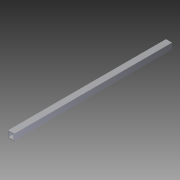
# Autodesk Inventor part: AB1-16-26-001
Saved by Autodesk Inventor 2011 SP1 (Build 150282100, 282)
## iProperties
Created: 2011-01-11
Part Number: AB1-16-26-001
Document SubType Name: Modeling
Designer: 12416547
Density: 1 g/cm^3
Author: 12416547
Autodesk Inventor part; units mm, degrees
ref_plane "YZ Plane" through (0, 0, 0) normal (1, 0, 0) x (0, 1, 0)
ref_plane "XZ Plane" through (0, 0, 0) normal (0, 1, 0) x (-1, 0, 0)
ref_plane "XY Plane" through (0, 0, 0) normal (0, 0, 1) x (1, 0, 0)
sketch "Sketch1" plane through (0, 0, 0) normal (0, 0, 1) x (1, 0, 0)
  line L0 (-24.2455, 20.5231) -> (1.1545, 20.5231)
  line L1 (1.1545, 20.5231) -> (1.1545, -4.8769)
  line L2 (1.1545, -4.8769) -> (-24.2455, -4.8769)
  line L3 (-24.2455, -4.8769) -> (-24.2455, 20.5231)
  line L4 (-0.433, 18.9356) -> (-22.658, 18.9356)
  line L5 (-22.658, 18.9356) -> (-22.658, -3.2894)
  line L6 (-22.658, -3.2894) -> (-0.433, -3.2894)
  line L7 (-0.433, -3.2894) -> (-0.433, 18.9356)
  point P0 (0, 0)
  dimension "d0" = 25.4
  dimension "d1" = 25.4
  dimension "d2" = 1.5875
  constraints: 16 end point, 4 parallel, 2 perpendicular, 1 horizontal, 3 other
  measures "d0" distance of L0.start L0.end
  measures "d1" distance of L2.end L0.start
  measures "d2" distance between parallel lines of L0 L4
extrude "Extrusion1" add sketch "Sketch1" against normal blind 660.4
body "Solid1"
